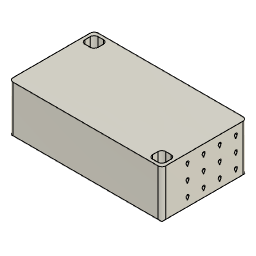
Assemblage (Autodesk Fusion 360 archive; units mm, degrees)
design "Haut"
Autodesk Fusion 360 part; units mm, degrees
ref_plane "WorkPlane1" through (39.5, 42.4, 4) normal (0, 0, 1) x (1, 0, 0)
sketch "Sketch1" plane through (0, 0, 4) normal (0, 0, 1) x (1, 0, 0)
  line L0 (1.6, 42.4) -> (77.4, 42.4)
  line L1 (1.6, 1.6) -> (1.6, 42.4)
  line L2 (77.4, 1.6) -> (1.6, 1.6)
  line L3 (77.4, 42.4) -> (77.4, 1.6)
ref_plane "WorkPlane2" through (79, 22, 5.6) normal (0, 0, 1) x (0, 1, 0)
extrude "Extrude1" add sketch "Sketch1" along normal up to surface (1.6 mm away)
ref_plane "WorkPlane3" through (74, 5, 4) normal (0, 0, 1) x (1, 0, 0)
sketch "Sketch3" plane through (0, 0, 4) normal (0, 0, 1) x (1, 0, 0)
  line L0 (75.6, 3.4) -> (72.4, 3.4)
  line L1 (72.4, 3.4) -> (72.4, 6.6)
  line L2 (72.4, 6.6) -> (75.6, 6.6)
  line L3 (75.6, 6.6) -> (75.6, 3.4)
  line L4 (6.6, 37.4) -> (3.4, 37.4)
  line L5 (3.4, 37.4) -> (3.4, 40.6)
  line L6 (3.4, 40.6) -> (6.6, 40.6)
  line L7 (6.6, 40.6) -> (6.6, 37.4)
  line L8 (77.4, 8.4) -> (77.4, 1.6)
  line L9 (77.4, 1.6) -> (70.6, 1.6)
  line L10 (70.6, 1.6) -> (70.6, 8.4)
  line L11 (70.6, 8.4) -> (77.4, 8.4)
  line L12 (8.4, 35.6) -> (1.6, 35.6)
  line L13 (1.6, 35.6) -> (1.6, 42.4)
  line L14 (1.6, 42.4) -> (8.4, 42.4)
  line L15 (8.4, 42.4) -> (8.4, 35.6)
  dimension "d6" = -1.8
  dimension "d7" = -1.8
sketch "Sketch4" plane through (0, 0, 4) normal (0, 0, 1) x (1, 0, 0)
  line L0 (70.6, 1.6) -> (70.6, 8.4)
  line L1 (70.6, 8.4) -> (77.4, 8.4)
  line L2 (69, 1.6) -> (69, 10)
  line L3 (69, 10) -> (77.4, 10)
  line L4 (1.6, 35.6) -> (8.4, 35.6)
  line L5 (8.4, 35.6) -> (8.4, 42.4)
  line L6 (1.6, 34) -> (10, 34)
  line L7 (10, 34) -> (10, 42.4)
  line L8 (69, 1.6) -> (70.6, 1.6)
  line L9 (77.4, 10) -> (77.4, 8.4)
  line L10 (1.6, 35.6) -> (1.6, 34)
  line L11 (8.4, 42.4) -> (10, 42.4)
  dimension "d8" = -1.6
  dimension "d9" = 1.6
  constraint coincident L0.start L8.end
  constraint perpendicular L0 L8
  constraint coincident L1.end L9.end
  constraint perpendicular L1 L9
  constraint coincident L4.start L10.start
  constraint perpendicular L6 L10
  constraint coincident L5.end L11.start
  constraint perpendicular L7 L11
move_body "Move1" bodies 1 to x (1, 0, 0) y (0, 1, 0) z (0, 0, 1) at (0, 0, 24)
extrude "Extrude2" add sketch "Sketch4" along normal up to surface (24 mm away)
sketch "Sketch5" plane through (0, 0, 28) normal (0, 0, -1) x (1, 0, 0)
  line L0 (77.4, -10) -> (69, -10)
  line L1 (69, -10) -> (69, -1.6)
  line L2 (69, -1.6) -> (1.6, -1.6)
  line L3 (1.6, -1.6) -> (1.6, -34)
  line L4 (1.6, -34) -> (10, -34)
  line L5 (10, -34) -> (10, -42.4)
  line L6 (10, -42.4) -> (77.4, -42.4)
  line L7 (77.4, -42.4) -> (77.4, -10)
sketch "Sketch6" plane through (0, 0, 28) normal (0, 0, -1) x (1, 0, 0)
  line L0 (1.6, -42.4) -> (77.4, -42.4)
  line L1 (1.6, -1.6) -> (1.6, -42.4)
  line L2 (77.4, -1.6) -> (1.6, -1.6)
  line L3 (77.4, -42.4) -> (77.4, -1.6)
  line L4 (79, 0) -> (0, 0)
  line L5 (0, 0) -> (0, -44)
  line L6 (0, -44) -> (79, -44)
  line L7 (79, -44) -> (79, 0)
  dimension "d12" = 1.6
extrude "Extrude3" add sketch "Sketch6" along normal up to surface (-1.6 mm away) and the other way up to surface (-24 mm away)
sketch "Sketch7" plane through (0, 0, 4) normal (0, 0, -1) x (1, 0, 0)
  line L0 (10, -42.4) -> (10, -34)
  line L1 (10, -34) -> (1.6, -34)
  line L2 (1.6, -34) -> (1.6, -1.6)
  line L3 (1.6, -1.6) -> (69, -1.6)
  line L4 (69, -1.6) -> (69, -10)
  line L5 (69, -10) -> (77.4, -10)
  line L6 (77.4, -10) -> (77.4, -42.4)
  line L7 (77.4, -42.4) -> (10, -42.4)
  line L8 (77.4, -8.4) -> (70.6, -8.4)
  line L9 (70.6, -8.4) -> (70.6, -1.6)
  line L10 (70.6, -1.6) -> (77.4, -1.6)
  line L11 (77.4, -1.6) -> (77.4, -8.4)
  line L12 (0, -44) -> (79, -44)
  line L13 (79, -44) -> (79, 0)
  line L14 (79, 0) -> (0, 0)
  line L15 (0, 0) -> (0, -44)
  line L16 (8.4, -42.4) -> (1.6, -42.4)
  line L17 (1.6, -42.4) -> (1.6, -35.6)
  line L18 (1.6, -35.6) -> (8.4, -35.6)
  line L19 (8.4, -35.6) -> (8.4, -42.4)
extrude "Extrude4" cut sketch "Sketch7" against normal blind 46 contours L8 L9 L10 L11 | L16 L17 L18 L19
sketch "Sketch8" plane through (0, 0, 4) normal (0, 0, -1) x (1, 0, 0)
  line L0 (10, -42.4) -> (10, -34)
  line L1 (10, -34) -> (1.6, -34)
  line L2 (1.6, -34) -> (1.6, -1.6)
  line L3 (1.6, -1.6) -> (69, -1.6)
  line L4 (69, -1.6) -> (69, -10)
  line L5 (69, -10) -> (77.4, -10)
  line L6 (77.4, -10) -> (77.4, -42.4)
  line L7 (77.4, -42.4) -> (10, -42.4)
  line L8 (77.4, -8.4) -> (70.6, -8.4)
  line L9 (70.6, -8.4) -> (70.6, -1.6)
  line L10 (70.6, -1.6) -> (77.4, -1.6)
  line L11 (77.4, -1.6) -> (77.4, -8.4)
  line L12 (0, -44) -> (79, -44)
  line L13 (79, -44) -> (79, 0)
  line L14 (79, 0) -> (0, 0)
  line L15 (0, 0) -> (0, -44)
  line L16 (8.4, -42.4) -> (1.6, -42.4)
  line L17 (1.6, -42.4) -> (1.6, -35.6)
  line L18 (1.6, -35.6) -> (8.4, -35.6)
  line L19 (8.4, -35.6) -> (8.4, -42.4)
  line L20 (6.6, -37.4) -> (3.4, -37.4)
  line L21 (6.6, -40.6) -> (6.6, -37.4)
  line L22 (3.4, -40.6) -> (6.6, -40.6)
  line L23 (3.4, -37.4) -> (3.4, -40.6)
  line L24 (75.6, -6.6) -> (75.6, -3.4)
  line L25 (75.6, -3.4) -> (72.4, -3.4)
  line L26 (72.4, -3.4) -> (72.4, -6.6)
  line L27 (72.4, -6.6) -> (75.6, -6.6)
extrude "Extrude5" add sketch "Sketch8" against normal blind 1.5 contours L8 L9 L10 L11 | L16 L17 L18 L19
chamfer "Chamfer1" distance 1.6 angle 45 4 edges at (39.5, 44, 4) (79, 22, 4) (39.5, 0, 4) (0, 22, 4)
sketch "Sketch11" plane through (0, 0, 0) normal (-1, 0, 0) x (0, -1, 0)
  line L0 (0, 29.6) -> (-44, 29.6)
  line L1 (-44, 29.6) -> (-44, 5.6)
  line L2 (0, 5.6) -> (0, 29.6)
  line L3 (-14.995, 13.6) -> (-8.995, 13.6)
  line L4 (-8.995, 13.6) -> (-8.995, 5.6)
  line L5 (-8.995, 5.6) -> (-14.995, 5.6)
  line L6 (-14.995, 5.6) -> (-14.995, 13.6)
  line L7 (-44, 5.6) -> (0, 5.6)
  line L8 (-13.465, 4.65) -> (-13.465, -0.85)
  line L9 (-10.525, 4.65) -> (-10.525, -0.85)
  dimension "d44" = 8
  dimension "d45" = 6
  dimension "d46" = 1.53
  dimension "d47" = 1.53
  constraint horizontal L3
  constraint vertical L4
  constraint horizontal L5
  constraint vertical L6
  constraint collinear L5 L7
  measures "d44" distance of L3.start L5.end
  measures "d45" distance of L3.start L3.end
  measures "d46" horizontal distance of L5.end L8.start
  measures "d47" horizontal distance of L4.end L9.start
extrude "Extrude7" cut sketch "Sketch11" against normal blind 3 contours L3 L4 L5 L6 L7
sketch "Sketch12" plane through (0, 0, 0) normal (-1, 0, 0) x (0, -1, 0)
  line L0 (-8.995, 13.6) -> (-8.995, 5.6)
  line L1 (-14.995, 5.6) -> (-14.995, 13.6)
  line L2 (-14.995, 13.6) -> (-8.995, 13.6)
  line L3 (0, 29.6) -> (-44, 29.6)
  line L4 (-44, 29.6) -> (-44, 5.6)
  line L5 (0, 5.6) -> (0, 29.6)
  line L6 (-17.395, 6.5) -> (-32.395, 6.5)
  line L7 (-32.395, 6.5) -> (-32.395, 26.5)
  line L8 (-32.395, 26.5) -> (-17.395, 26.5)
  line L9 (-17.395, 26.5) -> (-17.395, 6.5)
  line L10 (-8.995, 5.6) -> (0, 5.6)
  line L11 (-44, 5.6) -> (-14.995, 5.6)
  dimension "d42" = 15
  dimension "d43" = 20
  dimension "d58" = 2.4
  dimension "d59" = 0.9
  constraint horizontal L6
  constraint vertical L7
  constraint horizontal L8
  constraint vertical L9
  measures "d42" distance of L6.start L6.end
  measures "d43" distance of L6.start L8.end
  measures "d58" horizontal distance of L1.start L6.start
  measures "d59" vertical distance of L1.start L6.start
extrude "Extrude8" cut sketch "Sketch12" against normal blind 5 contours L6 L7 L8 L9
sketch "Sketch13" plane through (79, 0, 0) normal (1, 0, 0) x (0, 1, 0)
  line L0 (44, 29.6) -> (0, 29.6)
  line L1 (0, 29.6) -> (0, 5.6)
  line L2 (44, 5.6) -> (44, 29.6)
  line L3 (12.6268, 25.0205) -> (13.2837, 23.5439)
  line L4 (13.2837, 23.5439) -> (13.9873, 24.9989)
  arc A0 (12.6268, 25.0205) -> (13.9873, 24.9989) centre (13.3121, 25.3254) cw
  line L5 (21.6171, 23.5439) -> (22.3206, 24.9989)
  arc A1 (20.9602, 25.0205) -> (22.3206, 24.9989) centre (21.6454, 25.3254) cw
  line L6 (20.9602, 25.0205) -> (21.6171, 23.5439)
  line L7 (29.9504, 23.5439) -> (30.6539, 24.9989)
  arc A2 (29.2935, 25.0205) -> (30.6539, 24.9989) centre (29.9787, 25.3254) cw
  line L8 (29.2935, 25.0205) -> (29.9504, 23.5439)
  line L9 (38.2837, 23.5439) -> (38.9873, 24.9989)
  arc A3 (37.6268, 25.0205) -> (38.9873, 24.9989) centre (38.3121, 25.3254) cw
  line L10 (37.6268, 25.0205) -> (38.2837, 23.5439)
  line L11 (13.2837, 16.0439) -> (13.9873, 17.4989)
  arc A4 (12.6268, 17.5205) -> (13.9873, 17.4989) centre (13.3121, 17.8254) cw
  line L12 (12.6268, 17.5205) -> (13.2837, 16.0439)
  line L13 (21.6171, 16.0439) -> (22.3206, 17.4989)
  arc A5 (20.9602, 17.5205) -> (22.3206, 17.4989) centre (21.6454, 17.8254) cw
  line L14 (20.9602, 17.5205) -> (21.6171, 16.0439)
  line L15 (29.9504, 16.0439) -> (30.6539, 17.4989)
  arc A6 (29.2935, 17.5205) -> (30.6539, 17.4989) centre (29.9787, 17.8254) cw
  line L16 (29.2935, 17.5205) -> (29.9504, 16.0439)
  line L17 (38.2837, 16.0439) -> (38.9873, 17.4989)
  arc A7 (37.6268, 17.5205) -> (38.9873, 17.4989) centre (38.3121, 17.8254) cw
  line L18 (37.6268, 17.5205) -> (38.2837, 16.0439)
  line L19 (13.2837, 8.5439) -> (13.9873, 9.9989)
  arc A8 (12.6268, 10.0205) -> (13.9873, 9.9989) centre (13.3121, 10.3254) cw
  line L20 (12.6268, 10.0205) -> (13.2837, 8.5439)
  line L21 (21.6171, 8.5439) -> (22.3206, 9.9989)
  arc A9 (20.9602, 10.0205) -> (22.3206, 9.9989) centre (21.6454, 10.3254) cw
  line L22 (20.9602, 10.0205) -> (21.6171, 8.5439)
  line L23 (29.9504, 8.5439) -> (30.6539, 9.9989)
  arc A10 (29.2935, 10.0205) -> (30.6539, 9.9989) centre (29.9787, 10.3254) cw
  line L24 (29.2935, 10.0205) -> (29.9504, 8.5439)
  line L25 (38.2837, 8.5439) -> (38.9873, 9.9989)
  arc A11 (37.6268, 10.0205) -> (38.9873, 9.9989) centre (38.3121, 10.3254) cw
  line L26 (37.6268, 10.0205) -> (38.2837, 8.5439)
  line L27 (0, 5.6) -> (44, 5.6)
  dimension "d32" = 1.5
  dimension "d35" = 25
  dimension "d36" = -15
  constraint tangent L4 A0
  constraint tangent L3 A0
  measures "d32" diameter of A0
extrude "Extrude9" cut sketch "Sketch13" against normal blind 15 contours L3 L4 A0 | L5 A1 L6 | L7 A2 L8 | L9 A3 L10 | L11 A4 L12 | L13 A5 L14 | L15 A6 L16 | L17 A7 L18 | L19 A8 L20 | L21 A9 L22 | L23 A10 L24 | L25 A11 L26
extrude "Extrude10" add 2 faces at (73.4667, 2.2, 5.5) (4.4667, 36.2, 5.5) along direction (0, 0, 1) blind 3.3
fillet "Fillet1" radius 2 4 edges at (0, 44, 17.6) (0, 0, 17.6) (79, 0, 17.6) (79, 44, 17.6)
fillet "Fillet2" radius 2 8 edges at (8.4, 35.6, 19.2) (1.6, 35.6, 19.2) (1.6, 42.4, 19.2) (8.4, 42.4, 19.2) (77.4, 8.4, 19.2) (77.4, 1.6, 19.2) (70.6, 1.6, 19.2) (70.6, 8.4, 19.2)
fillet "Fillet3" radius 2 2 edges at (10, 34, 16) (69, 10, 16)
fillet "Fillet4" radius 2 4 edges at (69, 1.6, 16) (77.4, 10, 16) (1.6, 34, 16) (10, 42.4, 16)
chamfer "Chamfer2" distance 7.5 angle 45 2 edges at (0.8, 17.395, 6.5) (0.8197, 32.395, 6.5)
